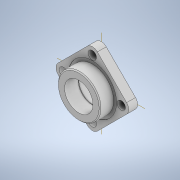
# Autodesk Inventor part: Деталь2
Saved by Autodesk Inventor 2021 (Build 250183000, 183)
## iProperties
Created: 2020-05-07
Part Number: Деталь2
Material: Типовые
Document SubType Name: Modeling
Designer: 2000
Density: 1 g/cm^3
Appearance: По умолчанию
Author: 2000
Autodesk Inventor part; units mm, degrees
ref_plane "YZ Plane" through (0, 0, 0) normal (1, 0, 0) x (0, 1, 0)
ref_plane "XZ Plane" through (0, 0, 0) normal (0, 1, 0) x (-1, 0, 0)
ref_plane "XY Plane" through (0, 0, 0) normal (0, 0, 1) x (1, 0, 0)
sketch "Эскиз1" plane through (0, 0, 0) normal (0, 0, 1) x (1, 0, 0)
  line L0 (-8.4853, 57.9828) -> (-57.9828, 8.4853)
  line L1 (-57.9828, -8.4853) -> (-8.4853, -57.9828)
  line L2 (8.4853, -57.9828) -> (57.9828, -8.4853)
  line L3 (57.9828, 8.4853) -> (8.4853, 57.9828)
  arc A0 (8.4853, 57.9828) -> (-8.4853, 57.9828) centre (0, 49.4975) ccw
  arc A1 (57.9828, -8.4853) -> (57.9828, 8.4853) centre (49.4975, 0) ccw
  arc A2 (-57.9828, 8.4853) -> (-57.9828, -8.4853) centre (-49.4975, 0) ccw
  arc A3 (-8.4853, -57.9828) -> (8.4853, -57.9828) centre (0, -49.4975) ccw
  point P0 (0, 0)
  point P1 (0, 66.468)
  point P2 (-66.468, 0)
  point P3 (0, -66.468)
  point P4 (66.468, 0)
  dimension "d0" = 94
  dimension "d1" = 47
  dimension "d2" = 47
  dimension "d3" = 12
  constraints: 8 end point, 8 point on circle, 8 point on line, 8 tangent, 4 centre point, 3 equal radius, 3 perpendicular, 1 horizontal alignment, 1 vertical alignment
  measures "d0" distance of point (66.468, 0) point (0, 66.468)
  measures "d1" distance from line of L3 point (0, 0)
  measures "d2" distance from line of point (0, 0) L2
  measures "d3" radius of A0
extrude "Выдавливание1" add sketch "Эскиз1" along normal blind 15
sketch "Эскиз2" plane through (0, 0, 15) normal (0, 0, 1) x (1, 0, 0)
  circle A0 centre (0, 0) radius 36
  dimension "d6" = 72
  constraints: 1 centre point, 1 coincident
  measures "d6" diameter of A0
extrude "Выдавливание2" add sketch "Эскиз2" along normal blind 23
sketch "Эскиз3" plane through (0, 0, 38) normal (0, 0, 1) x (1, 0, 0)
  circle A0 centre (0, 0) radius 24
  dimension "d9" = 48
  constraints: 1 centre point, 1 coincident
  measures "d9" diameter of A0
extrude "Выдавливание3" cut sketch "Эскиз3" against normal blind 38
chamfer "Фаска1" distance 1.6 angle 45 1 edges at (-36, 0, 38)
chamfer "Фаска2" distance 2 angle 45 1 edges at (-24, 0, 0)
sketch "Эскиз4" plane through (0, 0, 0) normal (0, 0, -1) x (-1, 0, 0)
  circle A0 centre (0, 49) radius 7
  circle A1 centre (49, 0) radius 7
  circle A2 centre (0, -49) radius 7
  circle A3 centre (-49, 0) radius 7
  line L0 (0, -86.0965) -> (0, 86.0965) projected
  line L1 (86.0965, 0) -> (-86.0965, 0) projected
  point P0 (0, 0)
  dimension "d18" = 98
  dimension "d19" = 98
  dimension "d20" = 14
  dimension "d21" = 14
  dimension "d22" = 14
  dimension "d23" = 14
  constraints: 4 centre point, 2 symmetric about line
  measures "d18" distance of A2.centre A0.centre
  measures "d19" distance of A3.centre A1.centre
  measures "d20" diameter of A0
  measures "d21" diameter of A1
  measures "d22" diameter of A3
  measures "d23" diameter of A2
extrude "Выдавливание4" cut sketch "Эскиз4" against normal blind 15
sketch "Эскиз5" plane through (0, 0, 15) normal (0, 0, 1) x (1, 0, 0)
  circle A0 centre (0, 0) radius 41
  dimension "d26" = 82
  constraints: 1 centre point, 1 coincident
  measures "d26" diameter of A0
extrude "Выдавливание5" cut sketch "Эскиз5" against normal blind 1
